Suction Adapter (Autodesk Fusion 360 design; units mm, degrees)
Autodesk Fusion 360 part; units mm, degrees
note: some values were not read from the file. Set by a fixed rule: which sketch regions a step uses.
sketch "Sketch2" plane through (0, 0, 0) normal (0, 1, 0) x (1, 0, 0)
  circle A0 centre (0, 0) radius 16.5
  circle A1 centre (0, 0) radius 17.5
  circle A2 centre (0, 0) radius 25.25
  circle A3 centre (0, 0) radius 27
  circle A4 centre (0, 0) radius 15.5
  circle A5 centre (0, 0) radius 13.5
  dimension "d6" = 33
  dimension "d11" = 35
  dimension "d29" = 50.5
  dimension "d37" = 54
  dimension "d41" = 31
  dimension "d42" = 27
  constraint coincident A0.centre A1.centre
  constraint concentric A3 A4
  measures "d6" diameter of A0
  measures "d11" diameter of A1
  measures "d29" diameter of A2
  measures "d37" diameter of A3
  measures "d41" diameter of A4
  measures "d42" diameter of A5
extrude "Extrude1" add sketch "Sketch2" along normal blind 31 contours A3
extrude "Extrude7" add sketch "Sketch2" along normal blind 3.5 from surface at 27.5 contours A1 | A2 | A3
extrude "Extrude4" add sketch "Sketch2" along normal blind 17 from surface at 31 contours A1
extrude "Extrude10" add sketch "Sketch2" along normal blind 40 from surface at 27 contours A0
extrude "Extrude11" add sketch "Sketch2" along normal blind 34 from surface at 45 contours A4
sketch "Sketch3" plane through (0, 0, 0) normal (1, 0, 0) x (0, 0, -1)
  ellipse E0 centre (0, 14.5) end of major axis (-6.75, 14.5) minor radius 4.5
  line L0 (6.75, 14.5) -> (-6.75, 14.5)
  line L1 (0, 19) -> (0, 10)
  dimension "d18" = 13.5
  dimension "d20" = 14.5
  dimension "d49" = 4.5
  constraint horizontal L0
  constraint coincident E0 L0.start
  constraint coincident E0 L0.end
  constraint coincident E0 L1.start
  constraint coincident E0 L1.end
  measures "d18" distance of E0
  measures "d20" distance of origin E0.centre
  measures "d49" distance of E0.centre L1.end
extrude "Extrude8" cut sketch "Sketch3" along normal mid plane 60
ref_plane "WorkPlane2" through (0, 27.5, 0) normal (0, -1, 0) x (-1, 0, 0)
chamfer "Chamfer1" distance 1 distance2 15 1 edges at (-16.3157, 48, 6.3283) measured on face at (17.0401, 48, 1.6891)
chamfer "Chamfer2" distance 1 distance2 5 1 edges at (-15.3834, 67, 5.9667) measured on face at (16.0475, 67, 1.5898)
